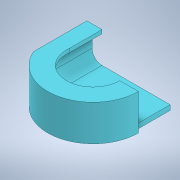
# Autodesk Inventor part: obudowa przekładni 5
Saved by Autodesk Inventor 2021 (Build 250183000, 183)
## iProperties
Created: 2022-01-26
Part Number: obudowa przekładni 5
Material: Generic
Document SubType Name: Modeling
Designer: Łukasz
Density: 1 g/cm^3
Appearance: Cadet Blue
Author: Łukasz
Autodesk Inventor part; units mm, degrees
ref_plane "YZ Plane" through (0, 0, 0) normal (1, 0, 0) x (0, 1, 0)
ref_plane "XZ Plane" through (0, 0, 0) normal (0, 1, 0) x (-1, 0, 0)
ref_plane "XY Plane" through (0, 0, 0) normal (0, 0, 1) x (1, 0, 0)
sketch "Sketch1" plane through (0, 0, 0) normal (0, 0, 1) x (1, 0, 0)
  line L0 (67, 4) -> (67, 0)
  line L1 (12.1369, 4) -> (67, 4)
  arc A0 (4.1369, 12) -> (12.1369, 4) centre (12.1369, 12) ccw
  line L2 (4.1369, 12) -> (4.1369, 32)
  line L3 (0, 0) -> (0, 32)
  line L4 (0, 0) -> (67, 0)
  line L5 (0, 32) -> (4.1369, 32)
  line L6 (0, 0) -> (0, 29)
  line L7 (0, 29) -> (4.1369, 29)
  line L8 (0, 26) -> (4.1369, 26)
  point P0 (53.5, 0)
  dimension "d13" = 29
  constraints: 18 end point, 4 point on line, 3 perpendicular, 2 point on circle, 1 centre point
  measures "d13" distance of L3.start L6.end
extrude "Extrusion1" add sketch "Sketch1" along normal blind 62 contours L0 L4 L3 L8 L2 A0 L1
sketch "Sketch2" plane through (0, 0, 0) normal (0, -1, 0) x (1, 0, 0)
  arc A0 (33.5, 62) -> (0, 28.5) centre (33.5, 28.5) ccw
  line L0 (0, 62) -> (67, 62) projected
  arc A1 (33.5, 65) -> (0, 42.9914) centre (33.5, 28.5) ccw
  line L1 (33.5, 62) -> (33.5, 65)
  line L2 (0, 0) -> (0, 62) projected
  line L3 (0, 28.5) -> (0, 42.9914)
  arc A2 (67, 28.5) -> (0, 28.5) centre (33.5, 28.5) ccw
  arc A3 (67, 14.0086) -> (0, 42.9914) centre (33.5, 28.5) ccw
  line L4 (67, 0) -> (67, 62) projected
  line L5 (67, 28.5) -> (70, 28.5)
  line L6 (67, 28.5) -> (70, 28.5) construction
  point P0 (47.9914, 62)
  point P1 (19.0086, 62)
  point P2 (67, 42.9914)
  dimension "d11" = 0
  constraints: 10 point on circle, 8 end point, 4 centre point, 4 point on line, 3 coincident, 2 midpoint, 1 collinear, 1 concentric, 1 horizontal, 1 perpendicular, 1 tangent
  measures "d11" distance between parallel lines of L5 L6
extrude "Extrusion2" add sketch "Sketch2" against normal blind 26 contours A0 L2 A1 L0 | L1 A3 L0 | L0 A1 L1 | L0 A3 L4 A2 | L4 A3 L5 picked at (67.5521, 36.6013)
sketch "Sketch3" plane through (0, 0, 0) normal (0, -1, 0) x (1, 0, 0)
  arc A0 (33.5, 65) -> (19.0086, 62) centre (33.5, 28.5) ccw projected
  circle A1 centre (33.5, 28.5) radius 33.5
  circle A2 centre (33.5, 28.5) radius 36.5
  line L0 (4.1369, 0) -> (4.1369, 44.6264) projected
  line L1 (0, 0) -> (0, 62) projected
  line L2 (47.9914, 62) -> (67, 62) projected
  line L3 (0, 0) -> (0, 62) projected
  line L4 (0, 0) -> (67, 0) projected
  line L5 (67, 42.9914) -> (67, 62) projected
  line L6 (47.9914, 62) -> (67, 62) projected
  arc A3 (70, 28.5) -> (67, 42.9914) centre (33.5, 28.5) ccw projected
  line L7 (0, 62) -> (19.0086, 62) projected
  arc A4 (47.9914, 62) -> (19.0086, 62) centre (33.5, 28.5) ccw projected
  line L8 (67, 0) -> (67, 28.5) projected
  line L9 (67, 28.5) -> (70, 28.5) projected
  point P0 (4.1369, 50.1809)
  point P1 (4.1369, 62)
  point P2 (33.5, 62)
  point P3 (19.0086, 62)
  point P4 (0, 42.9914)
  point P5 (47.9914, 62)
  point P6 (67, 42.9914)
  point P7 (33.5, 62)
  point P8 (47.9914, 62)
  point P9 (0, 42.9914)
  point P10 (0, 14.0086)
  point P11 (10.6965, 0)
  point P12 (56.3035, 0)
  point P13 (67, 42.9914)
  point P14 (19.0086, 62)
  point P15 (0, 28.5)
  point P16 (33.5, 62)
  point P17 (47.9914, 62)
  point P18 (51.1068, 0)
  point P19 (15.8932, 0)
  point P20 (70, 28.5)
  point P21 (67, 14.0086)
  point P22 (47.9914, 62)
  point P23 (19.0086, 62)
  constraints: 2 coincident, 4 other
extrude "Extrusion3" cut sketch "Sketch3" against normal blind 62 contours A2 L1 L7 | L2 L5 A2
ref_plane "Work Plane1" through (0, 32, 42.9914) normal (0, 1, 0) x (1, 0, 0)
sketch "Sketch5" plane through (0, 32, 42.9914) normal (0, 1, 0) x (1, 0, 0)
  arc A0 (0, 0) -> (70, 14.4914) centre (33.5, 14.4914) ccw projected
  line L0 (70, 14.4914) -> (55, 14.4914) projected
  arc A1 (12.1369, 16.914) -> (55, 14.4914) centre (33.5, 14.4914) ccw projected
  line L1 (12.1369, 16.914) -> (12.1369, 42.9914) projected
  line L2 (12.1369, 42.9914) -> (0, 42.9914) projected
  line L3 (0, 42.9914) -> (0, 0) projected
sketch "Sketch7" plane through (0, 26, 0) normal (0, 1, 0) x (1, 0, 0)
  arc A0 (0, -42.9914) -> (70, -28.5) centre (33.5, -28.5) ccw projected
  line L0 (70, -28.5) -> (55, -28.5) projected
  arc A1 (12.1369, -26.0774) -> (55, -28.5) centre (33.5, -28.5) ccw projected
  line L1 (12.1369, -26.0774) -> (12.1369, 0) projected
  line L2 (12.1369, 0) -> (0, 0) projected
  line L3 (0, 0) -> (0, -42.9914) projected
extrude "Extrusion6" add sketch "Sketch7" along normal blind 3
body "Solid1"
